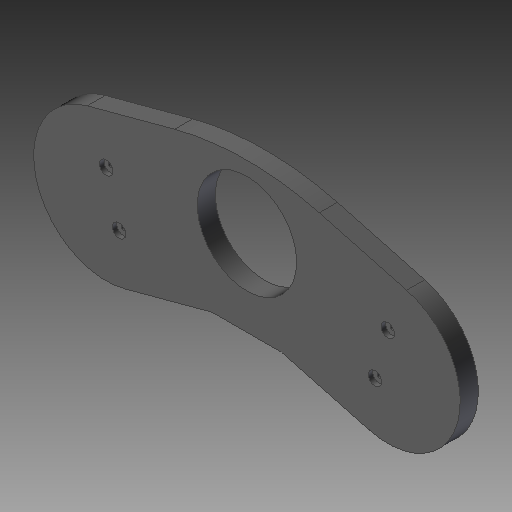
# Autodesk Inventor part: HA002
Saved by Autodesk Inventor 2017 SP1 (Build 210196100, 196)
## iProperties
Created: 2017-06-10
Part Number: HA002
Material: ABS Plastic
Document SubType Name: Modeling
Designer: Zach
Density: 1.06 g/cm^3
Appearance: CR White
Author: Zach
Autodesk Inventor part; units mm, degrees
ref_plane "YZ Plane" through (0, 0, 0) normal (1, 0, 0) x (0, 1, 0)
ref_plane "XZ Plane" through (0, 0, 0) normal (0, 1, 0) x (-1, 0, 0)
ref_plane "XY Plane" through (0, 0, 0) normal (0, 0, 1) x (1, 0, 0)
sketch "Sketch1" plane through (0, 0, 0) normal (0, 0, 1) x (1, 0, 0)
  line L0 (0, 0) -> (160, 0)
  line L1 (160, 0) -> (118.589, -154.5481)
  line L2 (0, 0) -> (41.411, -154.5481)
  line L3 (41.411, -154.5481) -> (118.589, -154.5481)
  dimension "d0" = 160
  dimension "d1" = 160
  dimension "d2" = 160
  dimension "d3" = 75
  dimension "d4" = 75
  constraints: 8 end point, 1 coincident, 1 horizontal
  measures "d0" distance of L0.start L0.end
  measures "d1" distance of L0.end L1.end
  measures "d2" distance of L0.start L2.end
  measures "d3" angle of L0 L1
  measures "d4" angle of L0 L2
extrude "Extrusion1" add sketch "Sketch1" along normal blind 20
sketch "Sketch5" plane through (0, 0, 20) normal (0, 0, 1) x (1, 0, 0)
  line L0 (160, 0) -> (0, 0) projected
  line L1 (160, 0) -> (256.5926, -25.8819)
  line L2 (118.589, -154.5481) -> (41.411, -154.5481) projected
  line L3 (118.589, -154.5481) -> (215.1815, -180.43)
  circle A0 centre (235.8871, -103.156) radius 80 construction
  arc A1 (215.1815, -180.43) -> (256.5926, -25.8819) centre (235.8871, -103.156) ccw
  line L4 (160, 0) -> (118.589, -154.5481)
  line L5 (0, 0) -> (41.411, -154.5481) projected
  line L6 (0, 0) -> (-96.5926, -25.8819)
  line L7 (41.411, -154.5481) -> (118.589, -154.5481) projected
  line L8 (41.411, -154.5481) -> (-55.1815, -180.43)
  circle A2 centre (-75.8871, -103.156) radius 80 construction
  arc A3 (-96.5926, -25.8819) -> (-55.1815, -180.43) centre (-75.8871, -103.156) ccw
  point P0 (90, 0)
  dimension "d25" = 100
  dimension "d26" = 100
  dimension "d27" = 160
  dimension "d30" = 100
  dimension "d31" = 100
  dimension "d32" = 160
  constraints: 10 end point, 8 point on circle, 6 tangent, 4 centre point, 1 concentric
  measures "d25" distance of L0.start L1.end
  measures "d26" distance of L2.start L3.end
  measures "d27" diameter of A0
  measures "d30" distance of L0.end L6.end
  measures "d31" distance of L2.end L8.end
  measures "d32" diameter of A2
extrude "Extrusion5" add sketch "Sketch5" against normal blind 20 contours L1 A1 L3 L4 | L5 L8 A3 L6
sketch "Sketch7" plane through (0, 0, 20) normal (0, 0, 1) x (1, 0, 0)
  line L0 (-75.7601, -74.6519) -> (-61.5251, -127.7778) construction
  line L1 (-68.6426, -101.2148) -> (20.7055, -77.2741) construction
  circle A0 centre (-75.7601, -74.6519) radius 2.5
  circle A1 centre (-61.5251, -127.7778) radius 2.5
  line L2 (0, 0) -> (-96.5926, -25.8819) construction
  line L3 (-55.1815, -180.43) -> (41.411, -154.5481) construction
  line L4 (-96.5926, -25.8819) -> (0, 0) construction
  line L5 (0, 0) -> (41.411, -154.5481) construction
  line L6 (41.411, -154.5481) -> (-55.1815, -180.43) construction
  line L7 (160, 0) -> (256.5926, -25.8819) construction
  line L8 (215.1815, -180.43) -> (118.589, -154.5481) construction
  line L9 (118.589, -154.5481) -> (160, 0) construction
  line L10 (139.2945, -77.2741) -> (228.6426, -101.2148) construction
  line L11 (221.5251, -127.7778) -> (235.7601, -74.6519) construction
  circle A2 centre (235.7601, -74.6519) radius 2.5
  circle A3 centre (221.5251, -127.7778) radius 2.5
  dimension "d35" = 55
  dimension "d37" = 5
  dimension "d38" = 5
  dimension "d46" = 92.5
  dimension "d47" = 92.5
  dimension "d48" = 55
  dimension "d49" = 5
  dimension "d50" = 5
  constraints: 12 end point, 6 perpendicular, 4 centre point, 4 coincident, 4 midpoint, 1 point on line
  measures "d35" distance of L0.start L0.end
  measures "d37" diameter of A0
  measures "d38" diameter of A1
  measures "d46" distance of L1.end L1.start
  measures "d47" distance of L10.end L10.start
  measures "d48" distance of L11.start L11.end
  measures "d49" diameter of A2
  measures "d50" diameter of A3
extrude "Extrusion7" cut sketch "Sketch7" against normal through all
sketch "Sketch8" plane through (0, 0, 20) normal (0, 0, 1) x (1, 0, 0)
  circle A0 centre (-75.7601, -74.6519) radius 2.5 projected
  circle A1 centre (-61.5251, -127.7778) radius 2.5 projected
  circle A2 centre (-75.7601, -74.6519) radius 7.5
  circle A3 centre (-61.5251, -127.7778) radius 7.5
  circle A4 centre (235.7601, -74.6519) radius 2.5 projected
  circle A5 centre (221.5251, -127.7778) radius 2.5 projected
  circle A6 centre (235.7601, -74.6519) radius 7.5
  circle A7 centre (221.5251, -127.7778) radius 7.5
  point P0 (0, 0)
  dimension "d42" = 15
  dimension "d43" = 15
  dimension "d51" = 15
  dimension "d52" = 15
  constraints: 4 centre point, 4 coincident
  measures "d42" diameter of A2
  measures "d43" diameter of A3
  measures "d51" diameter of A6
  measures "d52" diameter of A7
extrude "Extrusion8" cut sketch "Sketch8" against normal blind 5 contours A2 | A3 | A4 | A5 | A6 | A7
sketch "Sketch9" plane through (0, 0, 20) normal (0, 0, 1) x (1, 0, 0)
  circle A0 centre (80, -60) radius 55
  line L0 (41.411, -154.5481) -> (118.589, -154.5481) projected
  point P0 (0, 0)
  point P1 (80, -154.5481)
  dimension "d53" = 110
  dimension "d54" = 60
  constraints: 1 centre point, 1 midpoint, 1 vertical alignment
  measures "d53" diameter of A0
  measures "d54" vertical distance of A0.centre point (0, 0)
extrude "Extrusion9" cut sketch "Sketch9" against normal through all
sketch "Sketch10" plane through (0, 0, 20) normal (0, 0, 1) x (1, 0, 0)
  circle A0 centre (80, -304.672) radius 315 construction
  line L0 (160, 0) -> (0, 0) projected
  arc A1 (160, 0) -> (0, 0) centre (80, -304.672) ccw
  dimension "d57" = 630
  constraints: 4 point on circle, 2 centre point, 1 concentric
  measures "d57" diameter of A0
extrude "Extrusion10" add sketch "Sketch10" against normal blind 20
body "Solid1"
